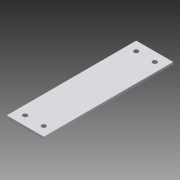
# Autodesk Inventor part: Battery Plate
Saved by Autodesk Inventor 2015 (Build 190159000, 159)
## iProperties
Created: 2015-02-07
Part Number: Battery Plate
Material: Aluminum 6061
Document SubType Name: Modeling
Designer: pltwe4
Density: 2.7 g/cm^3
Appearance: Aluminum - Flat
Author: pltwe4
Autodesk Inventor part; units mm, degrees
ref_plane "YZ Plane" through (0, 0, 0) normal (1, 0, 0) x (0, 1, 0)
ref_plane "XZ Plane" through (0, 0, 0) normal (0, 1, 0) x (-1, 0, 0)
ref_plane "XY Plane" through (0, 0, 0) normal (0, 0, 1) x (1, 0, 0)
sketch "Sketch1" plane through (0, 0, 0) normal (0, 1, 0) x (-1, 0, 0)
  line L0 (25.4, 88.9) -> (-25.4, 88.9)
  line L1 (-25.4, 88.9) -> (-25.4, -88.9)
  line L2 (-25.4, -88.9) -> (25.4, -88.9)
  line L3 (25.4, -88.9) -> (25.4, 88.9)
  line L4 (0, -124.46) -> (0, 124.46) projected
  line L5 (-35.56, 0) -> (35.56, 0) projected
  circle A0 centre (12.7, 76.2) radius 3.175
  circle A1 centre (12.7, -76.2) radius 3.175
  circle A2 centre (-12.7, -76.2) radius 3.175
  circle A3 centre (-12.7, 76.2) radius 3.175
  point P0 (0, 0)
  dimension "d0" = 50.8
  dimension "d1" = 177.8
  dimension "d6" = 6.35
  dimension "d7" = 12.7
  dimension "d8" = 12.7
  constraints: 8 end point, 4 centre point, 2 parallel, 1 horizontal, 1 perpendicular, 5 other
  measures "d0" distance between parallel lines of L1 L3
  measures "d1" distance of L2.end L0.start
  measures "d6" diameter of A0
  measures "d7" distance from line of L0 A0.centre
  measures "d8" distance from line of L4 A0.centre
extrude "Extrusion1" add sketch "Sketch1" along normal blind 3.175
body "Solid1"
